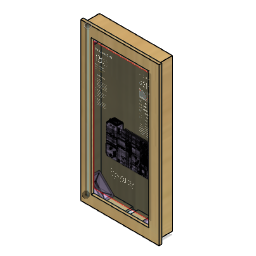
Smart Mirror (Autodesk Fusion 360 design; units mm, degrees)
Autodesk Fusion 360 part; units mm, degrees
sketch "Sketch1" plane through (0, 0, 0) normal (0, 1, 0) x (1, 0, 0)
  line L0 (0, 0) -> (150, 0)
  line L1 (150, 0) -> (150, -5)
  line L2 (150, -5) -> (0, -5)
  line L3 (0, -5) -> (0, 0)
  dimension "d1" = 150
  dimension "d2" = 5
  constraint horizontal L0
  constraint vertical L1
  constraint horizontal L2
  constraint vertical L3
  constraint coincident L0.start L3.end
  measures "d1" distance of L0.start L0.end
  measures "d2" distance of L0.start L2.end
extrude "Extrude1" add sketch "Sketch1" along normal blind 300 makes body 1
sketch "Sketch2" plane through (0, 0, 5) normal (0, 0, 1) x (1, 0, 0)
  line L0 (0, 0) -> (150, 0)
  line L1 (150, 0) -> (150, 300)
  line L2 (150, 300) -> (0, 300)
  line L3 (0, 300) -> (0, 0)
  line L4 (20, 280) -> (130, 280)
  line L5 (130, 280) -> (130, 20)
  line L6 (130, 20) -> (20, 20)
  line L7 (20, 20) -> (20, 280)
  constraint horizontal L4
  constraint vertical L5
  constraint horizontal L6
  constraint vertical L7
extrude "Extrude2" cut sketch "Sketch2" against normal blind 5 contours L4 L5 L6 L7 bodies 1
sketch "Sketch3" plane through (0, 0, 0) normal (0, 0, -1) x (-1, 0, 0)
  line L0 (-130, 20) -> (-130, 280)
  line L1 (-130, 280) -> (-20, 280)
  line L2 (-20, 280) -> (-20, 20)
  line L3 (-20, 20) -> (-130, 20)
  line L4 (-150, 0) -> (0, 0)
  line L5 (0, 0) -> (0, 300)
  line L6 (0, 300) -> (-150, 300)
  line L7 (-150, 300) -> (-150, 0)
  line L8 (-140, 290) -> (-10, 290)
  line L9 (-10, 290) -> (-10, 10)
  line L10 (-10, 10) -> (-140, 10)
  line L11 (-140, 10) -> (-140, 290)
  constraint horizontal L8
  constraint vertical L9
  constraint horizontal L10
  constraint vertical L11
extrude "Extrude3" cut sketch "Sketch3" along normal blind 1 contours L8 L9 L10 L11 bodies 1
ref_plane "WorkPlane1" through (75, 150, -0.5) normal (0, 0, -1) x (-1, 0, 0)
sketch "Sketch5" plane through (75, 150, -0.5) normal (0, 0, -1) x (1, 0, 0)
  line L0 (64.7738, -140.0467) -> (-64.0283, -140.0467)
  line L1 (-64.0283, -140.0467) -> (-64.0283, 138.5134)
  line L2 (-64.0283, 138.5134) -> (64.7738, 138.5134)
  line L3 (64.7738, 138.5134) -> (64.7738, -140.0467)
  constraint horizontal L0
  constraint vertical L1
  constraint horizontal L2
  constraint vertical L3
extrude "Extrude4" add sketch "Sketch5" along normal blind 1 separate body makes body 2
sketch "Sketch8" plane through (0, 0, 0) normal (0, 0, -1) x (-1, 0, 0)
  line L0 (-130, 20) -> (-130, 280)
  line L1 (-130, 280) -> (-20, 280)
  line L2 (-20, 280) -> (-20, 20)
  line L3 (-20, 20) -> (-130, 20)
  line L4 (-150, 0) -> (0, 0)
  line L5 (0, 0) -> (0, 300)
  line L6 (0, 300) -> (-150, 300)
  line L7 (-150, 300) -> (-150, 0)
  line L8 (-144.5555, 297.0382) -> (-4.9599, 297.0382)
  line L9 (-4.9599, 297.0382) -> (-4.9599, 292.1796)
  line L10 (-4.9599, 292.1796) -> (-144.5555, 292.1796)
  line L11 (-144.5555, 292.1796) -> (-144.5555, 297.0382)
  constraint horizontal L8
  constraint vertical L9
  constraint horizontal L10
  constraint vertical L11
extrude "Extrude5" add sketch "Sketch8" along normal blind 10 contours L8 L9 L10 L11 bodies 1
sketch "Sketch11" plane through (0, 0, 0) normal (0, 0, -1) x (-1, 0, 0)
  line L0 (-144.5555, 292.1796) -> (-144.5555, 297.0382)
  line L1 (-144.5555, 297.0382) -> (-4.9599, 297.0382)
  line L2 (-4.9599, 297.0382) -> (-4.9599, 292.1796)
  line L3 (-4.9599, 292.1796) -> (-144.5555, 292.1796)
  line L4 (-130, 20) -> (-130, 280)
  line L5 (-130, 280) -> (-20, 280)
  line L6 (-20, 280) -> (-20, 20)
  line L7 (-20, 20) -> (-130, 20)
  line L8 (-150, 0) -> (0, 0)
  line L9 (0, 0) -> (0, 300)
  line L10 (0, 300) -> (-150, 300)
  line L11 (-150, 300) -> (-150, 0)
  line L12 (-144.5555, 292.1796) -> (-141, 292.1796)
  line L13 (-141, 292.1796) -> (-141, 6)
  line L14 (-141, 6) -> (-144.5555, 6)
  line L15 (-144.5555, 6) -> (-144.5555, 292.1796)
  constraint horizontal L12
  constraint vertical L13
  constraint horizontal L14
  constraint vertical L15
  constraint coincident L0.start L3.end
extrude "Extrude6" add sketch "Sketch11" along normal blind 10 contours L3 L12 L13 L14 L15 bodies 1
sketch "Sketch12" plane through (0, 0, 0) normal (0, 0, -1) x (-1, 0, 0)
  line L0 (-150, 0) -> (0, 0)
  line L1 (0, 0) -> (0, 300)
  line L2 (0, 300) -> (-150, 300)
  line L3 (-150, 300) -> (-150, 0)
  line L4 (-130, 20) -> (-130, 280)
  line L5 (-130, 280) -> (-20, 280)
  line L6 (-20, 280) -> (-20, 20)
  line L7 (-20, 20) -> (-130, 20)
  line L8 (-141, 292.1796) -> (-141, 6)
  line L9 (-141, 6) -> (-144.5555, 6)
  line L10 (-144.5555, 6) -> (-144.5555, 297.0382)
  line L11 (-144.5555, 297.0382) -> (-4.9599, 297.0382)
  line L12 (-4.9599, 297.0382) -> (-4.9599, 292.1796)
  line L13 (-4.9599, 292.1796) -> (-141, 292.1796)
  line L14 (-141, 9.8047) -> (-5.1372, 9.8047)
  line L15 (-5.1372, 9.8047) -> (-5.1372, 6)
  line L16 (-5.1372, 6) -> (-141, 6)
  line L17 (-141, 6) -> (-141, 9.8047)
  constraint horizontal L14
  constraint vertical L15
  constraint horizontal L16
  constraint vertical L17
  constraint coincident L8 L14.start
extrude "Extrude7" add sketch "Sketch12" along normal blind 10 contours L8 L14 L15 L16 L17 bodies 1
sketch "Sketch13" plane through (0, 0, 0) normal (0, 0, -1) x (-1, 0, 0)
  line L0 (-141, 9.8047) -> (-5.1372, 9.8047)
  line L1 (-5.1372, 9.8047) -> (-5.1372, 6)
  line L2 (-5.1372, 6) -> (-144.5555, 6)
  line L3 (-144.5555, 6) -> (-144.5555, 297.0382)
  line L4 (-144.5555, 297.0382) -> (-4.9599, 297.0382)
  line L5 (-4.9599, 297.0382) -> (-4.9599, 292.1796)
  line L6 (-4.9599, 292.1796) -> (-141, 292.1796)
  line L7 (-141, 292.1796) -> (-141, 9.8047)
  line L8 (-130, 20) -> (-130, 280)
  line L9 (-130, 280) -> (-20, 280)
  line L10 (-20, 280) -> (-20, 20)
  line L11 (-20, 20) -> (-130, 20)
  line L12 (-150, 0) -> (0, 0)
  line L13 (0, 0) -> (0, 300)
  line L14 (0, 300) -> (-150, 300)
  line L15 (-150, 300) -> (-150, 0)
  line L16 (-5.1372, 9.8047) -> (-9, 9.8047)
  line L17 (-9, 9.8047) -> (-9, 292.1796)
  line L18 (-9, 292.1796) -> (-5.1372, 292.1796)
  line L19 (-5.1372, 292.1796) -> (-5.1372, 9.8047)
  constraint horizontal L16
  constraint vertical L17
  constraint horizontal L18
  constraint vertical L19
  constraint coincident L0.end L1.start
  constraint coincident L6 L17.end
mesh "Mesh1" [no effect]
mesh "Mesh2" [no effect]
mesh "Mesh3" [no effect]
mesh "Mesh4" [no effect]
mesh "Mesh5" [no effect]
sketch "Sketch16" plane through (0, 6, 0) normal (0, -1, 0) x (1, 0, 0)
  line L0 (144.5555, 0) -> (5.1372, 0)
  line L1 (5.1372, 0) -> (5.1372, -10)
  line L2 (5.1372, -10) -> (144.5555, -10)
  line L3 (144.5555, -10) -> (144.5555, 0)
  line L4 (70, -10) -> (80, -10)
  line L5 (80, -10) -> (80, -5)
  line L6 (80, -5) -> (70, -5)
  line L7 (70, -5) -> (70, -10)
  constraint horizontal L4
  constraint vertical L5
  constraint horizontal L6
  constraint vertical L7
  constraint coincident L2 L4.start
extrude "Extrude9" cut sketch "Sketch16" along normal blind 5 and the other way blind 5 contours L2 L4 L5 L6 L7 bodies 1
sketch "Sketch17" plane through (0, 0, -1.5) normal (0, 0, -1) x (-1, 0, 0)
  line L0 (-139.7738, 11.4866) -> (-10.9717, 11.4866)
  line L1 (-10.9717, 11.4866) -> (-10.9717, 290.0467)
  line L2 (-10.9717, 290.0467) -> (-139.7738, 290.0467)
  line L3 (-139.7738, 290.0467) -> (-139.7738, 11.4866)
ref_plane "WorkPlane3" through (75.3728, 150.7667, -1.6) normal (0, 0, -1) x (-1, 0, 0)
sketch "Sketch18" plane through (75.3728, 150.7667, -1.6) normal (0, 0, -1) x (1, 0, 0)
  line L0 (20, -80) -> (-20, -80)
  line L1 (-20, -80) -> (-20, -40)
  line L2 (-20, -40) -> (20, -40)
  line L3 (20, -40) -> (20, -80)
  constraint horizontal L0
  constraint vertical L1
  constraint horizontal L2
  constraint vertical L3
extrude "Extrude10" add sketch "Sketch18" along normal blind 10 separate body makes body 3
sketch "Sketch19" plane through (0, 0, 5) normal (0, 0, 1) x (1, 0, 0)
  line L0 (130, 280) -> (130, 20)
  line L1 (130, 20) -> (20, 20)
  line L2 (20, 20) -> (20, 280)
  line L3 (20, 280) -> (130, 280)
  line L4 (0, 0) -> (150, 0)
  line L5 (150, 0) -> (150, 300)
  line L6 (150, 300) -> (0, 300)
  line L7 (0, 300) -> (0, 0)
  line L8 (19.7226, 285.4428) -> (129.7535, 285.4428)
  line L9 (129.7535, 285.4428) -> (129.7535, 283.085)
  line L10 (129.7535, 283.085) -> (19.7226, 283.085)
  line L11 (19.7226, 283.085) -> (19.7226, 285.4428)
  constraint horizontal L8
  constraint vertical L9
  constraint horizontal L10
  constraint vertical L11
extrude "Extrude11" add sketch "Sketch19" along normal blind 2 separate body contours L8 L9 L10 L11 makes body 4
move_face "OffsetFaces1" offset 10 1 faces at (96.8385, 295.4187, -10) on bodies 1
extrude "Extrude12" add sketch "Sketch13" along normal blind 10 contours L0 L6 L16 L17 L18 L19 bodies 1
extrude "Extrude13" add 1 faces at (6.4248, 102.6614, -10) along direction (0, 0, -1) blind 10 on bodies 1 bodies 1
extrude "Extrude14" add 1 faces at (52.8385, 295.4187, -20) along direction (0, 0, -1) blind 5 on bodies 1 bodies 1
ref_plane "WorkPlane4" through (74.7577, 151.5191, -25) normal (0, 0, -1) x (-1, 0, 0)
sketch "Sketch20" plane through (74.7577, 151.5191, -25) normal (0, 0, -1) x (1, 0, 0)
  line L0 (69.7978, -145.5191) -> (-69.6205, -145.5191)
  line L1 (-69.6205, -145.5191) -> (-69.6205, 145.5191)
  line L2 (-69.6205, 145.5191) -> (69.7978, 145.5191)
  line L3 (69.7978, 145.5191) -> (69.7978, -145.5191)
  point P0 (69.7978, -145.5191)
  point P1 (-69.6205, 145.5191)
  constraint horizontal L0
  constraint vertical L1
  constraint horizontal L2
  constraint vertical L3
  constraint coincident P1 L1.end
  constraint coincident P0 L0.start
extrude "Extrude15" add sketch "Sketch20" along normal blind 1 bodies 1
extrude "Extrude8" [suppressed]
sketch "Sketch14" plane through (0, 0, -0.5) normal (0, 0, 1) x (1, 0, 0)
  line L0 (10.9717, 11.4866) -> (139.7738, 11.4866)
  line L1 (139.7738, 11.4866) -> (139.7738, 290.0467)
  line L2 (139.7738, 290.0467) -> (10.9717, 290.0467)
  line L3 (10.9717, 290.0467) -> (10.9717, 11.4866)
  line L4 (20, 280) -> (130, 280)
  line L5 (130, 280) -> (130, 20)
  line L6 (130, 20) -> (20, 20)
  line L7 (20, 20) -> (20, 280)
  point P0 (20, 280)
  point P1 (130, 20)
  constraint horizontal L4
  constraint vertical L5
  constraint horizontal L6
  constraint vertical L7
  constraint coincident P1 L5.end
  constraint coincident P0 L4.start
ref_plane "WorkPlane2" through (75.3728, 150.7667, -2.5) normal (0, 0, -1) x (-1, 0, 0)
hidden bodies 2 3 4
